Autodesk Fusion 360 part; units mm, degrees
(part 2 of 2)
  spline S78 degree 3 poles (96.6317, 1.0977) (96.5309, -0.12) (96.5309, -0.12) (91.3543, -3.7382) knots 0 0 0 0 1 1 1 1
  spline S79 degree 3 poles (66.4037, 64.1161) (66.4873, 64.0282) (66.5727, 63.9382) (66.6602, 63.8462) knots 0.977487 0.977487 0.977487 0.977487 1 1 1 1
  spline S80 degree 3 poles (17.1695, -12.3143) (11.43, -13.7614) (11.43, -13.7614) (8.1062, -10.6528) knots 0 0 0 0 1 1 1 1
  spline S81 degree 5 poles (61.3139, 67.1474) (61.543, 67.054) (61.7667, 66.9429) (61.9857, 66.8166) (62.2008, 66.6781) (62.4132, 66.5304) knots -0.787793 -0.787793 -0.787793 -0.787793 -0.787793 -0.787793 -0.634509 -0.634509 -0.634509 -0.634509 -0.634509 -0.634509
  spline S82 degree 3 poles (63.815, -8.5166) (63.6388, -8.805) (63.4757, -9.0721) (63.3225, -9.3195) knots 0 0 0 0 0.073817 0.073817 0.073817 0.073817
  spline S83 degree 3 poles (49.9069, 50.8075) (49.9549, 51.9293) (50.0447, 53.5537) (50.1761, 55.9334) knots 0.68255 0.68255 0.68255 0.68255 1 1 1 1
  arc A10 (45.4903, -1.6028) -> (57.8039, 5.4968) centre (38.1194, 25.4096) ccw
  spline S84 degree 3 poles (71.4046, -1.9621) (68.7161, -2.6699) (68.7161, -2.6699) (64.2045, 2.9631) knots 0 0 0 0 1 1 1 1
  arc A11 (16.6762, 7.4043) -> (23.8031, 1.3463) centre (38.1194, 25.4096) ccw
  spline S85 degree 3 poles (61.6897, 1.0229) (66.2013, -4.6101) (66.2013, -4.6101) (63.815, -8.5166) knots 0 0 0 0 1 1 1 1
  spline S86 degree 3 poles (50.6068, -10.9909) (49.9164, -10.1608) (49.1804, -8.8875) (48.0559, -6.9419) knots 0.654402 0.654402 0.654402 0.654402 1 1 1 1
  spline S87 degree 3 poles (57.8039, 5.4968) (58.7272, 4.7217) (59.8218, 3.3551) (61.6897, 1.0229) knots 0.585967 0.585967 0.585967 0.585967 1 1 1 1
  spline S88 degree 3 poles (50.1761, 55.9334) (50.5903, 63.43) (50.5903, 63.43) (56.6837, 65.6825) knots 0 0 0 0 1 1 1 1
  spline S89 degree 3 poles (7.41, 2.1159) (8.8689, 7.2633) (9.425, 7.2752) (14.2969, 7.3796) knots 0.114158 0.114158 0.114158 0.114158 1 1 1 1
  arc A12 (63.3225, -9.3195) -> (56.1134, -8.9752) centre (59.5529, -12.6043) ccw
  spline S90 degree 3 poles (24.7591, -6.9132) (22.9089, -10.8671) (22.9089, -10.8671) (17.1695, -12.3143) knots 0 0 0 0 1 1 1 1
  spline S91 degree 3 poles (64.2045, 2.9631) (61.7403, 6.0398) (60.622, 7.436) (60.7321, 8.897) knots 0 0 0 0 0.5462 0.5462 0.5462 0.5462
  line L16 (99.8062, -42.4114) -> (92.8433, -37.4077)
  spline S92 degree 3 poles (44.7999, -8.9657) (44.9787, -9.2749) (45.1476, -9.5671) (45.3066, -9.8441) knots 0 0 0 0 0.054921 0.054921 0.054921 0.054921
  spline S93 degree 3 poles (102.9685, -30.4014) (105.2318, -35.5312) (105.2318, -35.5312) (103.464, -39.4115) knots 0 0 0 0 1 1 1 1
  spline S94 degree 3 poles (120.7933, -29.7506) (120.8665, -30.0412) (120.9227, -30.3359) (120.9586, -30.633) knots -0.573046 -0.573046 -0.573046 -0.573046 -0.483074 -0.483074 -0.483074 -0.483074
  spline S95 degree 3 poles (93.0411, 9.3034) (87.475, 14.3719) (87.475, 14.3719) (89.8328, 18.2178) knots 0 0 0 0 1 1 1 1
  spline S96 degree 3 poles (99.012, 20.6558) (103.4238, 19.7452) (104.9823, 19.4236) (105.7891, 18.399) knots 0 0 0 0 0.646755 0.646755 0.646755 0.646755
  spline S97 degree 3 poles (89.8328, 18.2178) (92.1906, 22.0637) (92.1906, 22.0637) (99.012, 20.6558) knots 0 0 0 0 1 1 1 1
  spline S98 degree 5 poles (45.3066, -9.8441) (45.2696, -9.8381) (44.672, -9.7434) (44.0718, -9.673) (43.4715, -9.6267) (42.8725, -9.6043) (42.3117, -9.6043) knots -0.106605 -0.106605 -0.106605 -0.106605 -0.106605 -0.106605 -0.1 0 0 0 0 0 0
  spline S99 degree 3 poles (92.8433, -37.4077) (92.7385, -37.3323) (92.634, -37.2568) (92.4251, -37.1051) (92.3209, -37.0291) (92.2169, -36.9527) knots -0.077437 -0.077437 -0.077437 -0.077437 -0.038718 -0.038718 0 0 0 0
  spline S100 degree 3 poles (36.0251, -4.1706) (41.546, -3.3359) (41.546, -3.3359) (44.7999, -8.9657) knots 0 0 0 0 1 1 1 1
  spline S101 degree 3 poles (-1.9885, 37.6171) (2.8369, 36.7019) (2.9173, 36.6073) (3.9157, 35.4326) knots 0.080531 0.080531 0.080531 0.080531 1 1 1 1
  spline S102 degree 3 poles (18.1448, -16.4934) (19.6511, -16.1136) (20.7621, -15.8335) (21.6593, -15.7352) knots 0 0 0 0 0.262443 0.262443 0.262443 0.262443
  spline S103 degree 3 poles (98.4059, 5.3942) (97.1598, 5.553) (95.7688, 6.8196) (93.0411, 9.3034) knots 0.509948 0.509948 0.509948 0.509948 1 1 1 1
  spline S104 degree 5 poles (109.3117, -16.2751) (109.3576, -16.3439) (109.8768, -17.1135) (110.4405, -17.8559) (111.0514, -18.568) (111.7124, -19.2472) (112.356, -19.8386) knots -0.219582 -0.219582 -0.219582 -0.219582 -0.219582 -0.219582 -0.2 0 0 0 0 0 0
  arc A13 (119.7038, -30.964) -> (107.0095, -29.4439) centre (112.95, -33.6) ccw
  spline S105 degree 3 poles (106.6537, -28.6408) (104.3904, -23.511) (104.3904, -23.511) (107.4692, -18.9538) knots 0 0 0 0 1 1 1 1
  spline S106 degree 3 poles (105.7419, -45.5957) (105.69, -45.3714) (105.69, -45.3714) (107.4578, -41.4911) knots 0 0 0 0 1 1 1 1
  spline S107 degree 5 poles (105.7891, 18.399) (105.6715, 18.264) (105.2459, 17.8077) (104.4211, 17.0919) (103.084, 16.1991) (101.6527, 15.3939) (100.4204, 14.6999) (99.6248, 14.2381) (99.2336, 14.0074) knots -0.681054 -0.681054 -0.681054 -0.681054 -0.681054 -0.681054 -0.6 -0.4 -0.2 0 0 0 0 0 0
  line L17 (112.356, -19.8386) -> (117.5581, -24.6191)
  line L18 (18.0268, -18.6) -> (14.8735, -18.5603)
  spline S108 degree 5 poles (30.3517, -9.6043) (30.0793, -9.6043) (29.686, -9.6066) (29.2816, -9.6124) (28.8684, -9.625) (28.4508, -9.6506) (28.3281, -9.6595) knots -1 -1 -1 -1 -1 -1 -0.9 -0.858551 -0.858551 -0.858551 -0.858551 -0.858551 -0.858551
  spline S109 degree 3 poles (12.9904, -18.5603) (13.839, -17.5791) (15.2738, -17.2173) (18.1448, -16.4934) knots 0.499776 0.499776 0.499776 0.499776 1 1 1 1
  line L19 (-1.9885, 17.6992) -> (-1.9885, 37.6171)
  line L20 (14.8735, -18.5603) -> (12.9904, -18.5603)
  spline S110 degree 5 poles (21.6593, -15.7352) (21.5143, -16.0153) (21.1826, -16.6229) (20.6229, -17.4886) (19.9479, -18.1539) (19.0997, -18.5146) (18.4006, -18.6) (18.0268, -18.6) knots -0.281693 -0.281693 -0.281693 -0.281693 -0.281693 -0.281693 -0.2 -0.1 0 0 0 0 0 0
  spline S111 degree 3 poles (28.3281, -9.6595) (28.4291, -9.4399) (28.538, -9.2073) (28.6541, -8.9591) knots 0.93722 0.93722 0.93722 0.93722 1 1 1 1
  spline S112 degree 3 poles (103.464, -39.4115) (102.3427, -41.8725) (101.9326, -42.7727) (99.8062, -42.4114) knots 0 0 0 0 0.634238 0.634238 0.634238 0.634238
  spline S113 degree 3 poles (28.6541, -8.9591) (30.5043, -5.0052) (30.5043, -5.0052) (36.0251, -4.1706) knots 0 0 0 0 1 1 1 1
  line L21 (42.3117, -9.6043) -> (30.3517, -9.6043)
  spline S114 degree 5 poles (106.8571, 35.4674) (106.9247, 34.8367) (107.0589, 33.4167) (107.2059, 31.2061) (107.2698, 28.9352) (107.2676, 26.6633) (107.2369, 25.0234) (107.2136, 24.1743) (107.212, 24.116) knots -0.9599 -0.9599 -0.9599 -0.9599 -0.9599 -0.9599 -0.8 -0.6 -0.4 -0.385252 -0.385252 -0.385252 -0.385252 -0.385252 -0.385252
  spline S115 degree 3 poles (86.5898, -26.31) (88.7803, -23.8663) (88.7803, -23.8663) (94.7427, -24.569) knots 0 0 0 0 1 1 1 1
  spline S116 degree 3 poles (85.5398, -31.7467) (85.5284, -31.7381) (85.517, -31.7296) (85.4944, -31.7123) (85.4831, -31.7035) (85.4719, -31.6948) knots -0.008547 -0.008547 -0.008547 -0.008547 -0.004273 -0.004273 0 0 0 0
  spline S117 degree 3 poles (84.8934, -31.1604) (84.4785, -28.6653) (84.8158, -28.289) (86.5898, -26.31) knots 0.190125 0.190125 0.190125 0.190125 1 1 1 1
  spline S118 degree 3 poles (85.4719, -31.6948) (85.2716, -31.538) (85.0754, -31.3514) (84.8934, -31.1604) knots -0.221556 -0.221556 -0.221556 -0.221556 -0.145751 -0.145751 -0.145751 -0.145751
  spline S119 degree 3 poles (94.7427, -24.569) (100.7052, -25.2716) (100.7052, -25.2716) (102.9685, -30.4014) knots 0 0 0 0 1 1 1 1
  spline S120 degree 3 poles (98.2527, 36.3246) (104.1613, 36.928) (105.4636, 37.0609) (106.8571, 35.4674) knots 0 0 0 0 0.779606 0.779606 0.779606 0.779606
  spline S121 degree 3 poles (92.2169, -36.9527) (91.0564, -36.101) (90.0319, -35.3022) (87.6932, -33.4422) (86.6409, -32.5893) (85.5398, -31.7467) knots -0.831954 -0.831954 -0.831954 -0.831954 -0.415967 -0.415967 0 0 0 0
  spline S122 degree 3 poles (107.212, 24.116) (105.9507, 22.2482) (104.7833, 22.4891) (99.4569, 23.5885) knots 0.219152 0.219152 0.219152 0.219152 1 1 1 1
  spline S123 degree 3 poles (99.4569, 23.5885) (92.6354, 24.9964) (92.6354, 24.9964) (91.6111, 30.2304) knots 0 0 0 0 1 1 1 1
  spline S124 degree 3 poles (106.0703, 42.0666) (105.1197, 40.0631) (103.6036, 39.9083) (98.1201, 39.3484) knots 0.276494 0.276494 0.276494 0.276494 1 1 1 1
  spline S125 degree 3 poles (105.1245, -5.439) (100.6191, -0.6703) (100.6191, -0.6703) (100.7199, 0.5474) knots 0 0 0 0 1 1 1 1
  spline S126 degree 3 poles (81.2628, 35.2832) (86.639, 34.732) (86.639, 34.732) (87.6634, 29.498) knots 0 0 0 0 1 1 1 1
  spline S127 degree 3 poles (102.036, 52.4502) (103.2068, 52.0908) (104.1636, 51.789) (104.9375, 51.5064) knots 0.046165 0.046165 0.046165 0.046165 0.218876 0.218876 0.218876 0.218876
  arc A14 (93.8717, 53.28) -> (102.036, 52.4502) centre (98.5582, 58.8116) ccw
  spline S128 degree 3 poles (91.6111, 30.2304) (90.5867, 35.4645) (90.5867, 35.4645) (90.6302, 35.5076) knots 0 0 0 0 1 1 1 1
  line L22 (104.9375, 51.5064) -> (106.0703, 42.0666)
  line L23 (105.4239, -5.7558) -> (105.1245, -5.439)
  spline S129 degree 5 poles (101.9476, 2.7303) (102.0027, 2.6864) (102.3883, 2.3771) (103.0822, 1.7897) (104.0104, 0.8787) (104.73, -0.1686) (105.1055, -1.3672) (105.1957, -2.2743) (105.2008, -2.7549) knots 0.366854 0.366854 0.366854 0.366854 0.366854 0.366854 0.4 0.6 0.8 1 1 1 1 1 1
  spline S130 degree 3 poles (86.33, 20.418) (83.9721, 16.5722) (83.9721, 16.5722) (82.2856, 16.0675) knots 0 0 0 0 1 1 1 1
  spline S131 degree 5 poles (105.2008, -2.7549) (105.2051, -3.1627) (105.2248, -3.7661) (105.2639, -4.3673) (105.3216, -4.966) (105.3973, -5.562) (105.4239, -5.7558) knots -0.895379 -0.895379 -0.895379 -0.895379 -0.895379 -0.895379 -0.8 -0.753928 -0.753928 -0.753928 -0.753928 -0.753928 -0.753928
  spline S132 degree 3 poles (82.2856, 16.0675) (80.599, 15.5628) (80.599, 15.5628) (74.7407, 18.7711) knots 0 0 0 0 1 1 1 1
  spline S133 degree 3 poles (100.7199, 0.5474) (100.7832, 1.3128) (100.8067, 1.5971) (101.9476, 2.7303) knots 0 0 0 0 0.628482 0.628482 0.628482 0.628482
  spline S134 degree 3 poles (95.2171, -20.8274) (89.2546, -20.1248) (89.2546, -20.1248) (88.6138, -15.1197) knots 0 0 0 0 1 1 1 1
  spline S135 degree 3 poles (90.6302, 35.5076) (90.6737, 35.5507) (90.6737, 35.5507) (98.2527, 36.3246) knots 0 0 0 0 1 1 1 1
  spline S136 degree 3 poles (74.7407, 18.7711) (68.8825, 21.9793) (68.8825, 21.9793) (68.5302, 23.6499) knots 0 0 0 0 1 1 1 1
  spline S137 degree 3 poles (68.5302, 23.6499) (68.1779, 25.3204) (68.1779, 25.3204) (72.0322, 30.5774) knots 0 0 0 0 1 1 1 1
  spline S138 degree 3 poles (93.1496, -6.4964) (98.3262, -2.8782) (98.3262, -2.8782) (102.8316, -7.6469) knots 0 0 0 0 1 1 1 1
  spline S139 degree 3 poles (98.1201, 39.3484) (90.5411, 38.5744) (90.5411, 38.5744) (92.0688, 46.8006) knots 0 0 0 0 1 1 1 1
  spline S140 degree 3 poles (87.6634, 29.498) (88.6878, 24.2639) (88.6878, 24.2639) (86.33, 20.418) knots 0 0 0 0 1 1 1 1
  spline S141 degree 3 poles (72.0322, 30.5774) (75.8866, 35.8345) (75.8866, 35.8345) (81.2628, 35.2832) knots 0 0 0 0 1 1 1 1
  spline S142 degree 3 poles (102.8316, -7.6469) (107.3371, -12.4157) (107.3371, -12.4157) (104.2583, -16.9729) knots 0 0 0 0 1 1 1 1
  spline S143 degree 3 poles (104.2583, -16.9729) (101.1795, -21.5301) (101.1795, -21.5301) (95.2171, -20.8274) knots 0 0 0 0 1 1 1 1
  spline S144 degree 3 poles (91.3543, -3.7382) (86.1777, -7.3564) (86.1777, -7.3564) (81.7545, -4.7511) knots 0 0 0 0 1 1 1 1
  spline S145 degree 3 poles (92.0688, 46.8006) (92.7162, 50.287) (93.0893, 52.2958) (93.8717, 53.28) knots 0 0 0 0 0.423817 0.423817 0.423817 0.423817
  spline S146 degree 3 poles (73.1306, 15.5427) (78.9888, 12.3345) (78.9888, 12.3345) (76.541, 5.54) knots 0 0 0 0 1 1 1 1
  spline S147 degree 3 poles (88.6892, 47.3871) (87.1616, 39.1609) (87.1616, 39.1609) (87.1181, 39.1178) knots 0 0 0 0 1 1 1 1
  spline S148 degree 3 poles (76.541, 5.54) (74.0931, -1.2544) (74.0931, -1.2544) (71.4046, -1.9621) knots 0 0 0 0 1 1 1 1
  spline S149 degree 3 poles (87.1181, 39.1178) (87.0746, 39.0747) (87.0746, 39.0747) (81.6983, 39.6259) knots 0 0 0 0 1 1 1 1
  spline S150 degree 3 poles (79.7791, 4.6487) (82.227, 11.4431) (82.227, 11.4431) (83.9136, 11.9478) knots 0 0 0 0 1 1 1 1
  spline S151 degree 3 poles (88.714, 58.2763) (90.2169, 55.6132) (90.2169, 55.6132) (88.6892, 47.3871) knots 0 0 0 0 1 1 1 1
  spline S152 degree 3 poles (81.6983, 39.6259) (76.3221, 40.1771) (76.3221, 40.1771) (73.7684, 44.6578) knots 0 0 0 0 1 1 1 1
  spline S153 degree 3 poles (72.756, 53.7554) (74.2974, 58.3724) (74.2974, 58.3724) (80.7542, 59.6559) knots 0 0 0 0 1 1 1 1
  spline S154 degree 3 poles (48.0559, -6.9419) (46.4474, -4.1591) (45.634, -2.7519) (45.4903, -1.6028) knots 0 0 0 0 0.494297 0.494297 0.494297 0.494297
  arc A15 (7.0084, -9.6077) -> (7.41, 2.1159) centre (2.95, -3.6) ccw
  arc A16 (54.3001, 48.2609) -> (49.9069, 50.8075) centre (38.1194, 25.4096) ccw
  spline S155 degree 3 poles (6.5202, 24.8369) (8.1365, 30.8144) (8.588, 32.4843) (11.09, 32.718) knots 0 0 0 0 0.720641 0.720641 0.720641 0.720641
  arc A17 (65.8941, 28.9547) -> (57.9256, 45.2014) centre (38.1194, 25.4096) ccw
  spline S156 degree 3 poles (8.1062, -10.6528) (7.6887, -10.2623) (7.3236, -9.9209) (7.0084, -9.6077) knots 0 0 0 0 0.125615 0.125615 0.125615 0.125615
  spline S157 degree 3 poles (24.9414, 52.6817) (25.3585, 51.9185) (25.7214, 51.2544) (26.0303, 50.6653) knots 0 0 0 0 0.12979 0.12979 0.12979 0.12979
  arc A18 (26.0303, 50.6653) -> (12.8489, 37.4678) centre (38.1194, 25.4096) ccw
  spline S158 degree 3 poles (21.7431, 57.7896) (22.6267, 56.9174) (23.4274, 55.4523) (24.9414, 52.6817) knots 0.528805 0.528805 0.528805 0.528805 1 1 1 1
  spline S159 degree 3 poles (69.0019, 55.1405) (67.4605, 50.5235) (67.4605, 50.5235) (59.0236, 49.0688) knots 0 0 0 0 1 1 1 1
  spline S160 degree 3 poles (69.0393, 32.6843) (67.6515, 30.7914) (66.7634, 29.5801) (65.8941, 28.9547) knots 0 0 0 0 0.36006 0.36006 0.36006 0.36006
  arc A19 (14.9097, 49.8352) -> (21.8805, 55.231) centre (16.95, 54.4) ccw
  spline S161 degree 3 poles (13.5893, 11.9086) (8.7257, 11.8082) (8.6395, 11.8999) (6.5034, 14.1733) knots 0.040369 0.040369 0.040369 0.040369 1 1 1 1
  arc A20 (9.977, 37.8639) -> (11.8949, 37.5725) centre (11.6726, 42.5676) ccw
  spline S162 degree 3 poles (59.3492, 45.448) (67.7861, 46.9027) (67.7861, 46.9027) (70.3398, 42.422) knots 0 0 0 0 1 1 1 1
  spline S163 degree 3 poles (12.8489, 37.4678) (12.501, 37.5043) (12.1842, 37.5389) (11.8949, 37.5725) knots 0.162935 0.162935 0.162935 0.162935 0.240632 0.240632 0.240632 0.240632
  spline S164 degree 3 poles (59.0236, 49.0688) (57.0076, 48.7212) (55.4734, 48.4567) (54.3001, 48.2609) knots 0 0 0 0 0.238951 0.238951 0.238951 0.238951
  spline S165 degree 3 poles (70.3398, 42.422) (72.8936, 37.9413) (72.8936, 37.9413) (69.0393, 32.6843) knots 0 0 0 0 1 1 1 1
  spline S166 degree 3 poles (9.977, 37.8639) (8.8927, 38.1064) (8.6224, 38.4245) (8.0443, 39.1046) knots 0.467626 0.467626 0.467626 0.467626 1 1 1 1
  spline S167 degree 3 poles (57.9256, 45.2014) (58.3711, 45.2793) (58.8451, 45.361) (59.3492, 45.448) knots 0.940247 0.940247 0.940247 0.940247 1 1 1 1
  spline S168 degree 3 poles (6.5034, 14.1733) (4.2775, 16.5422) (4.2775, 16.5422) (6.5202, 24.8369) knots 0 0 0 0 1 1 1 1
  arc A21 (11.09, 32.718) -> (13.5893, 11.9086) centre (38.1194, 25.4096) ccw
  arc A22 (7.3843, 40.4707) -> (10.1529, 51.1029) centre (4.19, 46.9791) ccw
  spline S169 degree 3 poles (10.1529, 51.1029) (10.2459, 51.4148) (10.336, 51.7162) (10.4232, 52.0075) knots 0.023821 0.023821 0.023821 0.023821 0.056482 0.056482 0.056482 0.056482
  spline S170 degree 3 poles (8.0443, 39.1046) (7.6623, 39.5541) (7.4147, 39.8454) (7.3843, 40.4707) knots 0 0 0 0 0.351825 0.351825 0.351825 0.351825
  circle A23 centre (38.1194, 25.4096) radius 22
  spline S171 degree 5 poles (10.4232, 52.0075) (10.5195, 51.9767) (10.892, 51.8497) (11.5323, 51.5815) (12.4292, 51.1168) (13.3158, 50.6172) (14.1114, 50.2047) (14.6434, 49.9543) (14.9097, 49.8352) knots -0.669309 -0.669309 -0.669309 -0.669309 -0.669309 -0.669309 -0.6 -0.4 -0.2 0 0 0 0 0 0
  spline S172 degree 5 poles (21.8805, 55.231) (21.8039, 55.6854) (21.7452, 56.1936) (21.7156, 56.707) (21.714, 57.2234) (21.7403, 57.7392) (21.7431, 57.7896) knots 0 0 0 0 0 0 0.2 0.221657 0.221657 0.221657 0.221657 0.221657 0.221657
  spline S173 degree 3 poles (66.6602, 63.8462) (70.5433, 59.7574) (70.5433, 59.7574) (69.0019, 55.1405) knots 0 0 0 0 1 1 1 1
  spline S174 degree 3 poles (23.8031, 1.3463) (26.6021, -2.9749) (26.4935, -3.2069) (24.7591, -6.9132) knots 0.062609 0.062609 0.062609 0.062609 1 1 1 1
  circle A24 centre (2.8925, -3.5519) radius 5.25
  circle A25 centre (4.1554, 46.9532) radius 5.25
  circle A26 centre (67.5181, -20.6561) radius 5.25
  circle A27 centre (98.4809, 58.7861) radius 5.25
  circle A28 centre (112.8622, -33.5829) radius 5.25
  dimension "d11" = 10.5
  dimension "d12" = 10.5
  dimension "d13" = 10.5
  dimension "d14" = 10.5
  dimension "d15" = 10.5
  measures "d11" diameter of A24
  measures "d12" diameter of A25
  measures "d13" diameter of A26
  measures "d14" diameter of A27
  measures "d15" diameter of A28
extrude "돌출6" add sketch "스케치7" along normal blind 2 separate body makes body 2
extrude "돌출7" cut sketch "스케치7" along normal blind 2 draft 45 contours A0 | A1 | A2 | A3 bodies 2
extrude "돌출8" add sketch "스케치7" along normal blind 1 contours A24 | A25 | A26 | A27 | A28 bodies 2
hidden bodies 1
named bodies: "나노 마그넷", "일반마그넷"
